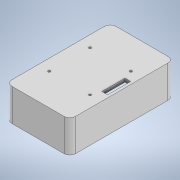
# Autodesk Inventor part: mount1
Saved by Autodesk Inventor 2020.2 (Build 242310000, 310)
## iProperties
Created: 2026-05-20
Part Number: mount1
Material: Generic
Document SubType Name: Modeling
Designer: explorer
Density: 1 g/cm^3
Appearance: Default
Author: explorer
Autodesk Inventor part; units mm, degrees
ref_plane "YZ Plane" through (0, 0, 0) normal (1, 0, 0) x (0, 1, 0)
ref_plane "XZ Plane" through (0, 0, 0) normal (0, 1, 0) x (-1, 0, 0)
ref_plane "XY Plane" through (0, 0, 0) normal (0, 0, 1) x (1, 0, 0)
sketch "Sketch1" plane through (0, 0, 0) normal (0, 1, 0) x (-1, 0, 0)
  line L0 (22.5, 45) -> (-22.5, 45)
  line L1 (-27.5, 40) -> (-27.5, -40)
  line L2 (-22.5, -45) -> (22.5, -45)
  line L3 (27.5, -40) -> (27.5, 40)
  line L4 (27.5, 45) -> (-27.5, -45) construction
  line L5 (-27.5, 45) -> (27.5, -45) construction
  line L6 (0, 0) -> (17.6777, 17.6777) construction
  line L7 (0, 0) -> (25, 0) construction
  circle A0 centre (17.6777, 17.6777) radius 1
  line L8 (17.6777, 17.6777) -> (21.2132, 14.1421) construction
  arc A1 (21.2132, 14.1421) -> (14.1421, 21.2132) centre (17.6777, 17.6777) ccw construction
  circle A2 centre (0, 0) radius 20 construction
  line L9 (14.1421, 21.2132) -> (10.1575, 17.2286) construction
  arc A3 (-6.25, 18.9984) -> (6.25, 18.9984) centre (0, 0) ccw construction
  line L10 (21.2132, 14.1421) -> (17.2286, 10.1575) construction
  line L11 (-14.1421, 21.2132) -> (-10.1575, 17.2286) construction
  arc A4 (-14.1421, 21.2132) -> (-21.2132, 14.1421) centre (-17.6777, 17.6777) ccw construction
  line L12 (-21.2132, 14.1421) -> (-17.2286, 10.1575) construction
  circle A5 centre (-17.6777, 17.6777) radius 1
  line L13 (-21.2132, -14.1421) -> (-17.2286, -10.1575) construction
  arc A6 (-21.2132, -14.1421) -> (-14.1421, -21.2132) centre (-17.6777, -17.6777) ccw construction
  line L14 (-14.1421, -21.2132) -> (-10.1575, -17.2286) construction
  circle A7 centre (-17.6777, -17.6777) radius 1
  line L15 (14.1421, -21.2132) -> (10.1575, -17.2286) construction
  arc A8 (14.1421, -21.2132) -> (21.2132, -14.1421) centre (17.6777, -17.6777) ccw construction
  line L16 (21.2132, -14.1421) -> (17.2286, -10.1575) construction
  circle A9 centre (17.6777, -17.6777) radius 1
  line L17 (-20.273, 10) -> (-25.273, 10)
  line L18 (-25.273, 10) -> (-25.273, -10)
  line L19 (-25.273, -10) -> (-20.273, -10)
  line L20 (-20.273, -10) -> (-20.273, 10)
  line L21 (-20.273, 10) -> (-25.273, -10) construction
  line L22 (-25.273, 10) -> (-20.273, -10) construction
  line L23 (39.9497, 0) -> (-39.9497, 0) projected
  arc A10 (22.5, -45) -> (27.5, -40) centre (22.5, -40) ccw
  arc A11 (27.5, 40) -> (22.5, 45) centre (22.5, 40) ccw
  arc A12 (-22.5, 45) -> (-27.5, 40) centre (-22.5, 40) ccw
  arc A13 (-27.5, -40) -> (-22.5, -45) centre (-22.5, -40) ccw
  point P0 (-22.773, 0)
  point P1 (-22.773, 0)
  dimension "d0" = 55
  dimension "d1" = 90
  dimension "d4" = 25
  dimension "d5" = 45
  dimension "d6" = 2
  dimension "d7" = 5
  dimension "d8" = 360
  dimension "d9" = 5
  dimension "d10" = 20
  dimension "d18" = 5
  constraints: 46 end point, 20 point on circle, 14 centre point, 10 point on line, 8 tangent, 6 parallel, 5 coincident, 5 midpoint, 3 equal radius, 3 horizontal, 3 perpendicular, 1 equal length, 41 other
  measures "d0" distance of L5.end L4.end
  measures "d1" distance of L4.end L5.start
  measures "d4" distance of L7.start L6.end
  measures "d5" angle of L7 L6
  measures "d6" diameter of A0
  measures "d7" distance of L8.start L10.start
  measures "d9" distance of L19.end L18.end
  measures "d10" distance of L18.end L17.end
  measures "d18" radius of A10
extrude "Extrusion1" add sketch "Sketch1" along normal blind 3 contours A11 L3 L23 L20 L17 L18 L1 A12 L0 | L3 A10 L2 A13 L1 L23 L18 L19 L20
sketch "Sketch2" plane through (0, 0, 0) normal (0, -1, 0) x (1, 0, 0)
  line L0 (22.5, 45) -> (-22.5, 45)
  line L1 (-27.5, 40) -> (-27.5, -40)
  line L2 (-22.5, -45) -> (22.5, -45)
  line L3 (27.5, -40) -> (27.5, 40)
  line L4 (27.5, 45) -> (-27.5, -45) construction
  line L5 (-27.5, 45) -> (27.5, -45) construction
  line L6 (17, 42.5) -> (-17, 42.5)
  line L7 (-25, 34.5) -> (-25, -34.5)
  line L8 (-17, -42.5) -> (17, -42.5)
  line L9 (25, -34.5) -> (25, 34.5)
  line L10 (25, 42.5) -> (-25, -42.5) construction
  line L11 (-25, 42.5) -> (25, -42.5) construction
  arc A0 (25, 34.5) -> (17, 42.5) centre (17, 34.5) ccw
  arc A1 (17, -42.5) -> (25, -34.5) centre (17, -34.5) ccw
  arc A2 (-25, -34.5) -> (-17, -42.5) centre (-17, -34.5) ccw
  arc A3 (-17, 42.5) -> (-25, 34.5) centre (-17, 34.5) ccw
  arc A4 (27.5, 40) -> (22.5, 45) centre (22.5, 40) ccw
  arc A5 (-22.5, 45) -> (-27.5, 40) centre (-22.5, 40) ccw
  arc A6 (-27.5, -40) -> (-22.5, -45) centre (-22.5, -40) ccw
  arc A7 (22.5, -45) -> (27.5, -40) centre (22.5, -40) ccw
  point P0 (0, 0)
  dimension "d13" = 55
  dimension "d14" = 90
  dimension "d15" = 50
  dimension "d16" = 85
  dimension "d17" = 8
  dimension "d21" = 5
  constraints: 24 end point, 16 point on circle, 16 point on line, 16 tangent, 8 centre point, 6 equal radius, 4 midpoint, 4 parallel, 2 horizontal, 2 perpendicular
  measures "d13" distance of L5.end L4.end
  measures "d14" distance of L4.end L5.start
  measures "d15" distance of L11.end L10.end
  measures "d16" distance of L10.end L11.start
  measures "d17" radius of A0
  measures "d21" radius of A4
extrude "Extrusion2" add sketch "Sketch2" along normal blind 25
body "Solid1"
